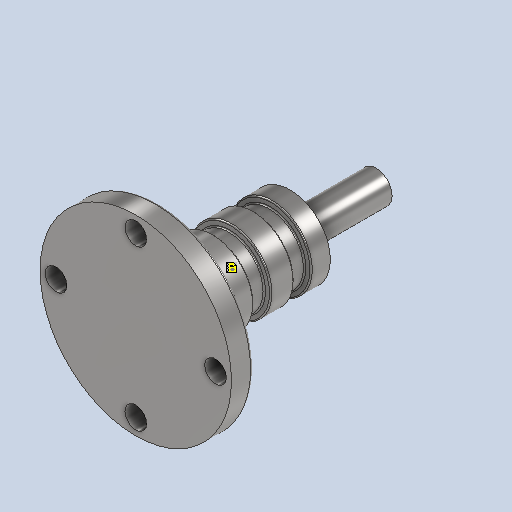
# Autodesk Inventor part: Rotor
Saved by Autodesk Inventor 2025.3 (Build 293356030, 356C)
## iProperties
Created: 2025-10-12
Part Number: Rotor
Material: Acero inoxidable
Document SubType Name: Modeling
Designer: santa
Density: 8 g/cm^3
Appearance: Semipulido
Author: santa
Autodesk Inventor part; units mm, degrees
ref_plane "YZ Plane" through (0, 0, 0) normal (1, 0, 0) x (0, 1, 0)
ref_plane "XZ Plane" through (0, 0, 0) normal (0, 1, 0) x (-1, 0, 0)
ref_plane "XY Plane" through (0, 0, 0) normal (0, 0, 1) x (1, 0, 0)
sketch "Boceto1" plane through (0, 0, 0) normal (0, 1, 0) x (-1, 0, 0)
  line L0 (0, 0) -> (-15, 0)
  line L1 (-15, 0) -> (-15, -3.5)
  line L2 (-15, -3.5) -> (-6.31, -3.5)
  line L3 (-6.31, -3.5) -> (-6.31, -12.194)
  line L4 (-6.31, -12.194) -> (-5.36, -12.2771)
  line L5 (-5.36, -12.2771) -> (-5.36, -14.7771)
  line L6 (-5.36, -14.7771) -> (-6.31, -14.8602)
  line L7 (-6.31, -14.8602) -> (-6.31, -18.5278)
  line L8 (-6.31, -18.5278) -> (-5.36, -18.6109)
  line L9 (-5.36, -18.6109) -> (-5.36, -21.1109)
  line L10 (-5.36, -21.1109) -> (-6.31, -21.194)
  line L11 (-6.31, -21.194) -> (-6.31, -24.194)
  line L12 (0, -37.694) -> (0, 0)
  line L13 (-5.36, -13.5271) -> (-6.26, -13.5271) construction
  line L14 (-5.36, -19.8609) -> (-6.1624, -19.8609) construction
  line L15 (-5.36, -12.2771) -> (-6.6407, -12.2771) construction
  line L16 (-6.81, -3.5) -> (-6.81, -24.194) construction
  line L17 (-6.31, -24.194) -> (-2.5, -24.194)
  line L18 (-2.5, -24.194) -> (-2.5, -37.694)
  line L19 (-2.5, -37.694) -> (0, -37.694)
  dimension "d0" = 30
  dimension "d1" = 3.5
  dimension "d3" = 2.5
  dimension "d4" = 5
  dimension "d6" = 0.5
  dimension "d7" = 8.694
  dimension "d9" = 3
  dimension "d10" = 5
  dimension "d11" = 13.5
  dimension "d33" = 20.694
  dimension "d36" = 13.62
  dimension "d37" = 1.45
  constraints: 40 end point, 7 point on line, 6 horizontal, 5 perpendicular, 2 equal length, 2 midpoint, 1 horizontal alignment, 1 parallel, 2 other
  measures "d0" diameter of L1 L12
  measures "d1" distance between parallel lines of L0 L2
  measures "d3" distance of L4.end L5.end
  measures "d4" angle of L4 L15
  measures "d6" distance between parallel lines of L3 L16
  measures "d7" distance of L2.end L3.end
  measures "d9" distance of L10.end L11.end
  measures "d10" diameter of L18 L12
  measures "d11" distance of L17.end L18.end
  measures "d33" distance between parallel lines of L2 L17
  measures "d36" diameter of L16 L12
  measures "d37" distance between parallel lines of L5 L16
revolve "Revolución1" add sketch "Boceto1" angle 360 about axis through (0, 0, -37.694) along (0, 0, 1)
fillet "Empalme1" radius 0.2 8 edges at (-6.31, 0, -21.194) (-5.36, 0, -21.1109) (-5.36, 0, -18.6109) (-6.31, 0, -18.5278) (-6.31, 0, -14.8602) (-5.36, 0, -14.7771) (-5.36, 0, -12.2771) (-6.31, 0, -12.194)
sketch "Boceto2" plane through (0, 0, -37.694) normal (0, 0, -1) x (-1, 0, 0)
  circle A0 centre (0, 0) radius 2.5 projected
  line L0 (1.5768, -1.94) -> (-1.5768, -1.94)
  point P0 (0, 0)
  point P1 (0, 2.5)
  point P2 (0, -1.94)
  dimension "d16" = 4.44
  constraints: 3 point on circle, 2 end point, 1 horizontal, 1 midpoint, 1 vertical alignment
  measures "d16" distance of point (0, 2.5) point (0, -1.94)
extrude "Extrusión1" cut sketch "Boceto2" against normal up to surface (13.5 mm away) contours L0 A0 picked at (-0.3662, -2.0419)
fillet "Empalme2" radius 0.5 1 edges at (-15, 0, -3.5)
sketch "Boceto3" plane through (0, 0, -3.5) normal (0, 0, -1) x (-1, 0, 0)
  point P0 (0, 0)
  point P1 (0, -12.5)
  point P2 (12.5, 0)
  point P3 (0, 12.5)
  point P4 (-12.5, 0)
  dimension "d20" = 12.5
  dimension "d23" = 360
  constraints: 1 vertical alignment, 5 other
  measures "d20" distance of point (0, 0) point (0, -12.5)
hole "Agujero1" at (0, -12.5, -3.5) at (-12.5, 0, -3.5) at (0, 12.5, -3.5) at (12.5, 0, -3.5) direction (0, 0, 1) diameter 3.4 end through all clearance for "Tornillo de cabeza plana avellanada ISO 2009/7046" size "M3" standard "ISO"
fillet "Empalme3" radius 2 1 edges at (-6.31, 0, -3.5)
fillet "Empalme4" radius 2 2 edges at (0, 2.5, -24.194) (0, -1.94, -24.194)
